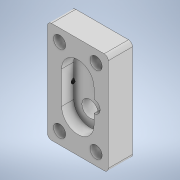
# Autodesk Inventor part: zad 7
Saved by Autodesk Inventor 2020 (Build 240168000, 168)
## iProperties
Created: 2022-03-14
Part Number: zad 7
Material: Ogólny
Document SubType Name: Modeling
Designer: 3IG
Density: 1 g/cm^3
Appearance: Domyślna
Author: 3IG
Autodesk Inventor part; units mm, degrees
ref_plane "YZ Plane" through (0, 0, 0) normal (1, 0, 0) x (0, 1, 0)
ref_plane "XZ Plane" through (0, 0, 0) normal (0, 1, 0) x (-1, 0, 0)
ref_plane "XY Plane" through (0, 0, 0) normal (0, 0, 1) x (1, 0, 0)
sketch "Szkic1" plane through (0, 0, 0) normal (0, 0, 1) x (1, 0, 0)
  line L0 (-1, 0) -> (-14, 0)
  line L1 (-15, 1) -> (-15, 24)
  line L2 (-14, 25) -> (-1, 25)
  line L3 (0, 24) -> (0, 1)
  arc A0 (-14, 25) -> (-15, 24) centre (-14, 24) ccw
  arc A1 (0, 24) -> (-1, 25) centre (-1, 24) ccw
  arc A2 (-1, 0) -> (0, 1) centre (-1, 1) ccw
  arc A3 (-15, 1) -> (-14, 0) centre (-14, 1) ccw
  circle A4 centre (-3, 3) radius 1.5
  circle A5 centre (-12, 3) radius 1.5
  circle A6 centre (-12, 22) radius 1.5
  circle A7 centre (-3, 22) radius 1.5
  circle A8 centre (-7.5, 8.5) radius 2
  circle A9 centre (-3.5, 12.5) radius 2.5
  point P0 (0, 0)
  point P1 (-15, 25)
  point P2 (-15, 0)
  point P3 (0, 25)
  point P4 (-11.5, 20.5)
  point P5 (-11.5, 4.5)
  point P6 (-3.5, 20.5)
  dimension "d0" = 15
  dimension "d1" = 25
  dimension "d2" = 1
  dimension "d3" = 3
  dimension "d4" = 3
  dimension "d5" = 3
  dimension "d6" = 3
  dimension "d7" = 8
  dimension "d8" = 16
  dimension "d10" = 19
  dimension "d11" = 4
  constraints: 10 centre point, 8 end point, 8 point on circle, 8 point on line, 8 tangent, 3 equal radius, 2 parallel, 1 horizontal, 1 perpendicular
  measures "d0" distance of point (-15, 25) point (0, 25)
  measures "d1" distance of point (-15, 0) point (-15, 25)
  measures "d2" radius of A0
  measures "d3" diameter of A4
  measures "d4" diameter of A5
  measures "d5" diameter of A6
  measures "d6" diameter of A7
  measures "d7" distance of point (-11.5, 20.5) point (-3.5, 20.5)
  measures "d8" distance of point (-11.5, 4.5) point (-11.5, 20.5)
  measures "d10" distance of A4.centre A7.centre
  measures "d11" diameter of A8
extrude "Wyciągnięcie proste2" add sketch "Szkic1" along normal blind 3
sketch "Szkic12" plane through (0, 0, 3) normal (0, 0, 1) x (1, 0, 0)
  line L0 (-1, 0) -> (-14, 0)
  line L1 (-15, 1) -> (-15, 24)
  line L2 (-14, 25) -> (-1, 25)
  line L3 (0, 24) -> (0, 1)
  arc A0 (-14, 25) -> (-15, 24) centre (-14, 24) ccw
  arc A1 (0, 24) -> (-1, 25) centre (-1, 24) ccw
  arc A2 (-1, 0) -> (0, 1) centre (-1, 1) ccw
  arc A3 (-15, 1) -> (-14, 0) centre (-14, 1) ccw
  circle A4 centre (-3, 3) radius 1.5
  circle A5 centre (-12, 3) radius 1.5
  circle A6 centre (-12, 22) radius 1.5
  circle A7 centre (-3, 22) radius 1.5
  circle A8 centre (-7.5, 8.5) radius 2
  circle A9 centre (-3.5, 12.5) radius 2.5
  line L4 (-7.5, 4.5) -> (-7.5, 4.5)
  line L5 (-11.5, 8.5) -> (-11.5, 16.5)
  line L6 (-7.5, 20.5) -> (-7.5, 20.5)
  line L7 (-3.5, 16.5) -> (-3.5, 8.5)
  arc A10 (-7.5, 20.5) -> (-11.5, 16.5) centre (-7.5, 16.5) ccw
  arc A11 (-3.5, 16.5) -> (-7.5, 20.5) centre (-7.5, 16.5) ccw
  arc A12 (-7.5, 4.5) -> (-3.5, 8.5) centre (-7.5, 8.5) ccw
  arc A13 (-11.5, 8.5) -> (-7.5, 4.5) centre (-7.5, 8.5) ccw
  arc A14 (-3.5, 11) -> (-3.5, 14) centre (-3.5, 12.5) ccw
  point P0 (0, 0)
  point P1 (0, 0)
  point P2 (-15, 25)
  point P3 (-15, 0)
  point P4 (0, 25)
  point P5 (-11.5, 20.5)
  point P6 (-11.5, 4.5)
  point P7 (-3.5, 20.5)
  point P8 (-11.5, 4.5)
  point P9 (-3.5, 20.5)
  dimension "d38" = 15
  dimension "d39" = 25
  dimension "d40" = 1
  dimension "d41" = 3
  dimension "d42" = 3
  dimension "d43" = 3
  dimension "d44" = 3
  dimension "d45" = 8
  dimension "d46" = 16
  dimension "d47" = 19
  dimension "d48" = 4
  dimension "d49" = 8
  dimension "d50" = 16
  dimension "d51" = 4
  dimension "d52" = 3
  constraints: 18 point on circle, 16 end point, 16 point on line, 16 tangent, 15 centre point, 6 equal radius, 4 parallel, 2 horizontal, 2 perpendicular, 1 coincident
  measures "d38" distance of point (-15, 25) point (0, 25)
  measures "d39" distance of point (-15, 0) point (-15, 25)
  measures "d40" radius of A0
  measures "d41" diameter of A4
  measures "d42" diameter of A5
  measures "d43" diameter of A6
  measures "d44" diameter of A7
  measures "d45" distance of point (-11.5, 20.5) point (-3.5, 20.5)
  measures "d46" distance of point (-11.5, 4.5) point (-11.5, 20.5)
  measures "d47" distance of A4.centre A7.centre
  measures "d48" diameter of A8
  measures "d49" distance of point (-11.5, 20.5) point (-3.5, 20.5)
  measures "d50" distance of point (-11.5, 4.5) point (-11.5, 20.5)
  measures "d51" radius of A10
  measures "d52" diameter of A14
extrude "Wyciągnięcie proste3" add sketch "Szkic12" along normal blind 3 contours L0 A3 L1 A0 L2 A1 L3 A2 | A9 L7 A14
sketch "Szkic16" plane through (-15, 1, 0) normal (-1, 0, 0) x (0, 0, 1)
  circle A0 centre (3, 11.5) radius 2.5
  line L0 (0, 14) -> (0, 9) projected
  point P0 (0, -1)
  dimension "d55" = 5
  constraints: 1 centre point
  measures "d55" diameter of A0
hole "Otwór2" at (-15, 12.5, 3) direction (1, 0, 0) diameter 5 depth 1.5 tip angle 118
sketch "Szkic17" plane through (-15, 1, 0) normal (-1, 0, 0) x (0, 0, 1)
  line L0 (3, 14) -> (3, 9) projected
  circle A0 centre (3, 11.5) radius 1.5
  point P0 (0, -1)
  dimension "d64" = 3
  constraints: 1 centre point, 1 midpoint
  measures "d64" diameter of A0
hole "Otwór3" at (-15, 12.5, 3) direction (1, 0, 0) diameter 3 depth 3 tip angle 118
